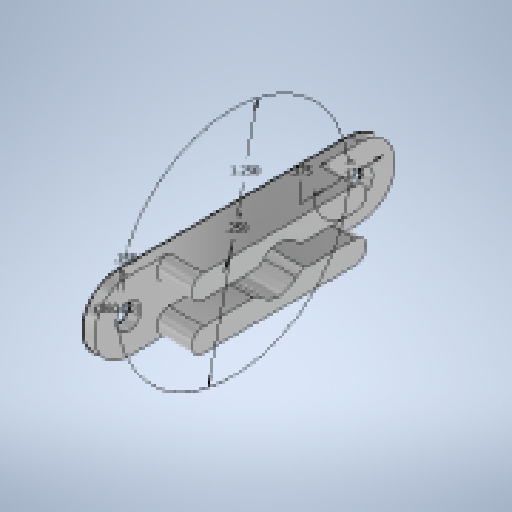
# Autodesk Inventor part: Pin Slot
Saved by Autodesk Inventor 2023.2 (Build 272271000, 271)
## iProperties
Created: 2024-01-24
Part Number: Pin Slot
Material: Aluminum 6061
Document SubType Name: Modeling
Designer: Nathan Cai
Density: 2.7 g/cm^3
Appearance: Aluminum - Flat
Author: Nathan Cai
Autodesk Inventor part; units mm, degrees
ref_plane "YZ Plane" through (0, 0, 0) normal (1, 0, 0) x (0, 1, 0)
ref_plane "XZ Plane" through (0, 0, 0) normal (0, 1, 0) x (-1, 0, 0)
ref_plane "XY Plane" through (0, 0, 0) normal (0, 0, 1) x (1, 0, 0)
sketch "Sketch1" plane through (0, 0, 0) normal (1, 0, 0) x (0, 1, 0)
  circle A0 centre (0, 0) radius 3.175
  circle A1 centre (0, 0) radius 15.875 construction
  line L0 (0, 0) -> (0, 15.875) construction
  circle A2 centre (0, 15.875) radius 1.7526
  circle A3 centre (0, -15.875) radius 1.7526
  line L1 (0, 15.875) -> (0, -15.875) construction
  line L2 (-4.7625, 15.875) -> (-4.7625, -15.875)
  line L3 (4.7625, -15.875) -> (4.7625, 15.875)
  arc A4 (4.7625, 15.875) -> (-4.7625, 15.875) centre (0, 15.875) ccw
  arc A5 (-4.7625, -15.875) -> (4.7625, -15.875) centre (0, -15.875) ccw
  line L4 (1.5875, 15.1324) -> (-1.5875, 15.1324) construction
  line L5 (-1.5875, 15.1324) -> (-1.5875, -15.1324)
  line L6 (-1.5875, -15.1324) -> (1.5875, -15.1324) construction
  line L7 (1.5875, -15.1324) -> (1.5875, 15.1324)
  line L8 (1.5875, 15.1324) -> (-1.5875, -15.1324) construction
  line L9 (-1.5875, 15.1324) -> (1.5875, -15.1324) construction
  circle A6 centre (0, 15.875) radius 4.7625
  circle A7 centre (0, -15.875) radius 4.7625
  point P0 (-4.7625, -15.875)
  point P1 (-1.5875, -11.3849)
  point P2 (-1.5875, -2.7496)
  point P3 (-1.5875, 2.7496)
  point P4 (-1.5875, 11.3849)
  point P5 (1.5875, 11.3849)
  point P6 (1.5875, 2.7496)
  point P7 (1.5875, -2.7496)
  point P8 (1.5875, -11.3849)
  dimension "d1" = 31.75
  dimension "d0" = 6.35
  dimension "d2" = 3.5052
  dimension "d5" = 360
  dimension "d7" = 9.525
  dimension "d8" = 3.175
  constraints: 22 end point, 5 coincident, 4 centre point, 4 point on circle, 4 tangent, 3 midpoint, 3 parallel, 2 vertical, 1 horizontal, 1 perpendicular, 1 vertical alignment, 16 other
  measures "d0" diameter of A0
  measures "d2" diameter of A2
  measures "d7" diameter of A5
  measures "d8" distance of L6.end L5.end
extrude "Extrusion1" add sketch "Sketch1" along normal blind 1.5875 contours A0 L7 A6 L3 A7 | A0 L5 A6 L7 | L7 A7 L5 A0 | A0 L5 A7 L2 A6 | A6 L5 A2 L7 | L7 A2 L5 A6 A4 | A7 A5 L5 A3 L7 | L7 A3 L5 A7
extrude "Extrusion2" add sketch "Sketch1" along normal blind 6.35 contours A0 L7 A6 L3 A7 | A0 L5 A7 L2 A6
fillet "Fillet1" radius 1.5875 8 edges at (3.9687, 4.7625, 15.875) (3.9687, -4.7625, 15.875) (3.9687, 4.7625, -15.875) (3.9687, -4.7625, -15.875) (3.9687, 1.5875, -11.3849) (3.9687, -1.5875, -11.3849) (3.9687, 1.5875, 11.3849) (3.9687, -1.5875, 11.3849)
fillet "Fillet2" radius 1.5875 4 edges at (3.9687, 1.5875, 2.7496) (3.9687, -1.5875, 2.7496) (3.9687, 1.5875, -2.7496) (3.9687, -1.5875, -2.7496)
body "Solid1"
